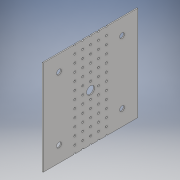
# Autodesk Inventor part: Drill Jig Base
Saved by Autodesk Inventor 2018 (Build 220112000, 112)
## iProperties
Created: 2018-12-05
Part Number: Drill Jig Base
Material: Generic
Document SubType Name: Modeling
Designer: gbgic
Density: 1 g/cm^3
Appearance: Default
Author: gbgic
Autodesk Inventor part; units mm, degrees
ref_plane "YZ Plane" through (0, 0, 0) normal (1, 0, 0) x (0, 1, 0)
ref_plane "XZ Plane" through (0, 0, 0) normal (0, 1, 0) x (-1, 0, 0)
ref_plane "XY Plane" through (0, 0, 0) normal (0, 0, 1) x (1, 0, 0)
sketch "Sketch1" plane through (0, 0, 0) normal (1, 0, 0) x (0, 1, 0)
  line L0 (4.9868, 295.4813) -> (-299.8132, 295.4813)
  line L1 (-299.8132, 295.4813) -> (-299.8132, -9.3187)
  line L2 (-299.8132, -9.3187) -> (4.9868, -9.3187)
  line L3 (4.9868, -9.3187) -> (4.9868, 295.4813)
  point P0 (0, 0)
  dimension "d0" = 304.8
  dimension "d1" = 304.8
  constraints: 8 end point, 2 parallel, 1 horizontal, 1 perpendicular
  measures "d0" distance of L2.end L1.end
  measures "d1" distance of L0.end L1.end
extrude "Extrusion1" add sketch "Sketch1" along normal blind 3.175
sketch "Sketch2" plane through (3.175, 0, 0) normal (1, 0, 0) x (0, 0, -1)
  line L0 (-143.0813, 4.9868) -> (-143.0813, -147.4132)
  circle A0 centre (-143.0813, -147.4132) radius 12.7
  point P0 (0, 0)
  point P1 (9.3187, 4.9868)
  dimension "d4" = 152.4
  dimension "d5" = 25.4
  constraints: 2 end point, 1 centre point, 1 coincident
  measures "d4" distance of L0.start L0.end
  measures "d5" diameter of A0
extrude "Extrusion2" cut sketch "Sketch2" against normal blind 50.8
sketch "Sketch3" plane through (3.175, 0, 0) normal (1, 0, 0) x (0, 0, -1)
  circle A0 centre (-143.0813, -147.4132) radius 12.7 projected
  circle A1 centre (-143.0813, -122.0132) radius 3.175
  circle A2 centre (-143.0813, -96.6132) radius 3.175
  circle A3 centre (-143.0813, -71.2132) radius 3.175
  circle A4 centre (-143.0813, -45.8132) radius 3.175
  circle A5 centre (-143.0813, -20.4132) radius 3.175
  circle A6 centre (-143.0813, 4.9868) radius 3.175
  line L0 (9.3187, -299.8132) -> (9.3187, 4.9868) projected
  circle A7 centre (-143.0813, -172.8132) radius 3.175
  circle A8 centre (-143.0813, -198.2132) radius 3.175
  circle A9 centre (-143.0813, -249.0132) radius 3.175
  circle A10 centre (-143.0813, -223.6132) radius 3.175
  circle A11 centre (-143.0813, -299.8132) radius 3.175
  circle A12 centre (-143.0813, -274.4132) radius 3.175
  circle A13 centre (-168.4813, -122.0132) radius 3.175
  circle A14 centre (-168.4813, -96.6132) radius 3.175
  circle A15 centre (-168.4813, -45.8132) radius 3.175
  circle A16 centre (-168.4813, -71.2132) radius 3.175
  circle A17 centre (-168.4813, 4.9868) radius 3.175
  circle A18 centre (-168.4813, -20.4132) radius 3.175
  circle A19 centre (-168.4813, -299.8132) radius 3.175
  circle A20 centre (-168.4813, -249.0132) radius 3.175
  circle A21 centre (-168.4813, -274.4132) radius 3.175
  circle A22 centre (-168.4813, -223.6132) radius 3.175
  circle A23 centre (-168.4813, -198.2132) radius 3.175
  circle A24 centre (-168.4813, -172.8132) radius 3.175
  circle A25 centre (-117.6813, -122.0132) radius 3.175
  circle A26 centre (-117.6813, -96.6132) radius 3.175
  circle A27 centre (-117.6813, -45.8132) radius 3.175
  circle A28 centre (-117.6813, -71.2132) radius 3.175
  circle A29 centre (-117.6813, 4.9868) radius 3.175
  circle A30 centre (-117.6813, -20.4132) radius 3.175
  circle A31 centre (-117.6813, -299.8132) radius 3.175
  circle A32 centre (-117.6813, -249.0132) radius 3.175
  circle A33 centre (-117.6813, -274.4132) radius 3.175
  circle A34 centre (-117.6813, -223.6132) radius 3.175
  circle A35 centre (-117.6813, -198.2132) radius 3.175
  circle A36 centre (-117.6813, -172.8132) radius 3.175
  circle A37 centre (-193.8813, -122.0132) radius 3.175
  circle A38 centre (-193.8813, -96.6132) radius 3.175
  circle A39 centre (-193.8813, -45.8132) radius 3.175
  circle A40 centre (-193.8813, -71.2132) radius 3.175
  circle A41 centre (-193.8813, 4.9868) radius 3.175
  circle A42 centre (-193.8813, -20.4132) radius 3.175
  circle A43 centre (-193.8813, -299.8132) radius 3.175
  circle A44 centre (-193.8813, -249.0132) radius 3.175
  circle A45 centre (-193.8813, -274.4132) radius 3.175
  circle A46 centre (-193.8813, -223.6132) radius 3.175
  circle A47 centre (-193.8813, -198.2132) radius 3.175
  circle A48 centre (-193.8813, -172.8132) radius 3.175
  circle A49 centre (-92.2813, -122.0132) radius 3.175
  circle A50 centre (-92.2813, -96.6132) radius 3.175
  circle A51 centre (-92.2813, -45.8132) radius 3.175
  circle A52 centre (-92.2813, -71.2132) radius 3.175
  circle A53 centre (-92.2813, 4.9868) radius 3.175
  circle A54 centre (-92.2813, -20.4132) radius 3.175
  circle A55 centre (-92.2813, -299.8132) radius 3.175
  circle A56 centre (-92.2813, -249.0132) radius 3.175
  circle A57 centre (-92.2813, -274.4132) radius 3.175
  circle A58 centre (-92.2813, -223.6132) radius 3.175
  circle A59 centre (-92.2813, -198.2132) radius 3.175
  circle A60 centre (-92.2813, -172.8132) radius 3.175
  point P0 (0, 0)
  dimension "d9" = 6.35
  dimension "d11" = 6.35
  dimension "d12" = 6.35
  dimension "d13" = 6.35
  dimension "d14" = 6.35
  dimension "d15" = 6.35
  dimension "d18" = 6.35
  dimension "d19" = 6.35
  dimension "d20" = 6.35
  dimension "d21" = 6.35
  dimension "d22" = 6.35
  dimension "d23" = 6.35
  dimension "d24" = 6.35
  dimension "d25" = 6.35
  dimension "d26" = 6.35
  dimension "d27" = 6.35
  dimension "d28" = 6.35
  dimension "d29" = 6.35
  dimension "d33" = 6.35
  dimension "d35" = 6.35
  dimension "d36" = 6.35
  dimension "d37" = 6.35
  dimension "d38" = 6.35
  dimension "d39" = 6.35
  dimension "d41" = 6.35
  dimension "d43" = 6.35
  dimension "d44" = 6.35
  dimension "d45" = 6.35
  dimension "d46" = 6.35
  dimension "d47" = 6.35
  constraints: 60 centre point
  measures "d9" diameter of A1
  measures "d11" diameter of A2
  measures "d12" diameter of A3
  measures "d13" diameter of A4
  measures "d14" diameter of A5
  measures "d15" diameter of A6
  measures "d18" diameter of A13
  measures "d19" diameter of A14
  measures "d20" diameter of A16
  measures "d21" diameter of A15
  measures "d22" diameter of A18
  measures "d23" diameter of A17
  measures "d24" diameter of A25
  measures "d25" diameter of A26
  measures "d26" diameter of A28
  measures "d27" diameter of A27
  measures "d28" diameter of A30
  measures "d29" diameter of A29
  measures "d33" diameter of A37
  measures "d35" diameter of A38
  measures "d36" diameter of A40
  measures "d37" diameter of A39
  measures "d38" diameter of A42
  measures "d39" diameter of A41
  measures "d41" diameter of A49
  measures "d43" diameter of A50
  measures "d44" diameter of A52
  measures "d45" diameter of A51
  measures "d46" diameter of A54
  measures "d47" diameter of A53
extrude "Extrusion3" cut sketch "Sketch3" against normal blind 50.8
sketch "Sketch4" plane through (3.175, 0, 0) normal (1, 0, 0) x (0, 0, -1)
  circle A0 centre (-143.0813, -147.4132) radius 12.7 projected
  line L0 (-143.0813, -147.4132) -> (-117.6813, -147.4132)
  line L1 (-117.6813, -147.4132) -> (-92.2813, -147.4132)
  circle A1 centre (-92.2813, -147.4132) radius 3.175
  circle A2 centre (-117.6813, -147.4132) radius 3.175
  circle A3 centre (-193.8813, -147.4132) radius 3.175
  circle A4 centre (-168.4813, -147.4132) radius 3.175
  point P0 (0, 0)
  dimension "d54" = 25.4
  dimension "d55" = 25.4
  dimension "d56" = 6.35
  dimension "d57" = 6.35
  constraints: 4 centre point, 4 end point, 2 coincident, 1 horizontal, 1 point on line
  measures "d54" distance of L0.start L0.end
  measures "d55" distance of L0.end L1.end
  measures "d56" diameter of A1
  measures "d57" diameter of A2
extrude "Extrusion4" cut sketch "Sketch4" against normal blind 50.8 contours A1 | A2 L1 L0 | L0 L1 A2 | A3 | A4
sketch "Sketch5" plane through (3.175, 0, 0) normal (1, 0, 0) x (0, 0, -1)
  line L0 (-295.4813, 4.9868) -> (-295.4813, -299.8132) projected
  circle A0 centre (-244.6813, -249.0132) radius 7.9375
  circle A1 centre (-41.4813, -249.0132) radius 7.9375
  line L1 (-244.6813, -249.0132) -> (-244.6813, -45.8132) construction
  circle A2 centre (-244.6813, -45.8132) radius 7.9375
  circle A3 centre (-41.4813, -45.8132) radius 7.9375
  point P0 (0, 0)
  dimension "d63" = 15.875
  dimension "d67" = 203.2
  dimension "d69" = 15.875
  dimension "d70" = 15.875
  constraints: 4 centre point, 2 end point, 1 coincident, 1 vertical
  measures "d63" diameter of A0
  measures "d67" distance of L1.start L1.end
  measures "d69" diameter of A2
  measures "d70" diameter of A3
extrude "Extrusion5" cut sketch "Sketch5" against normal blind 914.4
body "Solid1"
